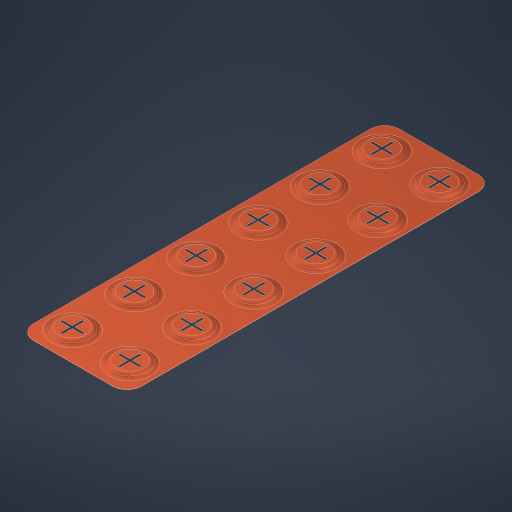
# Autodesk Inventor part: Bat_contacts_v1
Saved by Autodesk Inventor 2024.3 (Build 283343010, 343A)
## iProperties
Created: 2025-05-07
Part Number: Bat_contacts_v1
Material: Kupfer
Document SubType Name: Sheet Metal
Designer: David
Density: 8.94 g/cm^3
Appearance: Kupfer - satiniert
Sheet Metal Rule: Standard_mm
Author: David
Autodesk Inventor part; units mm, degrees
ref_plane "YZ Plane" through (0, 0, 0) normal (1, 0, 0) x (0, 1, 0)
ref_plane "XZ Plane" through (0, 0, 0) normal (0, 1, 0) x (-1, 0, 0)
ref_plane "XY Plane" through (0, 0, 0) normal (0, 0, 1) x (1, 0, 0)
sketch "Skizze1" plane through (0, 0, 0) normal (0, 0, 1) x (1, 0, 0)
  circle A0 centre (-20, 119.25) radius 9
  circle A1 centre (-20, 76.25) radius 9
  circle A2 centre (-20, 33.25) radius 9
  circle A3 centre (-20, 11.75) radius 9
  circle A4 centre (-20, 54.75) radius 9
  circle A5 centre (-20, 97.75) radius 9
  circle A6 centre (-40, 119.25) radius 9
  circle A7 centre (-40, 76.25) radius 9
  circle A8 centre (-40, 33.25) radius 9
  circle A9 centre (-40, 11.75) radius 9
  circle A10 centre (-40, 54.75) radius 9
  circle A11 centre (-40, 97.75) radius 9
  circle A12 centre (-20, 11.75) radius 9
  circle A13 centre (-20, 76.25) radius 9
  circle A14 centre (-20, 76.25) radius 9
  line L0 (-48.75, 129) -> (-11.25, 129)
  line L1 (-11.25, 129) -> (-11.25, 2)
  line L2 (-11.25, 2) -> (-48.75, 2)
  line L3 (-48.75, 2) -> (-48.75, 129)
  line L4 (-25, 16.75) -> (-15, 16.75)
  line L5 (-15, 16.75) -> (-15, 6.75)
  line L6 (-15, 6.75) -> (-25, 6.75)
  line L7 (-25, 6.75) -> (-25, 16.75)
  line L8 (-45, 16.75) -> (-35, 16.75)
  line L9 (-45, 6.75) -> (-45, 16.75)
  line L10 (-35, 6.75) -> (-45, 6.75)
  line L11 (-35, 16.75) -> (-35, 6.75)
  line L12 (-25, 38.25) -> (-15, 38.25)
  line L13 (-25, 28.25) -> (-25, 38.25)
  line L14 (-15, 28.25) -> (-25, 28.25)
  line L15 (-15, 38.25) -> (-15, 28.25)
  line L16 (-45, 38.25) -> (-35, 38.25)
  line L17 (-45, 28.25) -> (-45, 38.25)
  line L18 (-35, 28.25) -> (-45, 28.25)
  line L19 (-35, 38.25) -> (-35, 28.25)
  line L20 (-25, 59.75) -> (-15, 59.75)
  line L21 (-25, 49.75) -> (-25, 59.75)
  line L22 (-15, 49.75) -> (-25, 49.75)
  line L23 (-15, 59.75) -> (-15, 49.75)
  line L24 (-45, 59.75) -> (-35, 59.75)
  line L25 (-45, 49.75) -> (-45, 59.75)
  line L26 (-35, 49.75) -> (-45, 49.75)
  line L27 (-35, 59.75) -> (-35, 49.75)
  line L28 (-25, 81.25) -> (-15, 81.25)
  line L29 (-25, 71.25) -> (-25, 81.25)
  line L30 (-15, 71.25) -> (-25, 71.25)
  line L31 (-15, 81.25) -> (-15, 71.25)
  line L32 (-45, 81.25) -> (-35, 81.25)
  line L33 (-45, 71.25) -> (-45, 81.25)
  line L34 (-35, 71.25) -> (-45, 71.25)
  line L35 (-35, 81.25) -> (-35, 71.25)
  line L36 (-25, 102.75) -> (-15, 102.75)
  line L37 (-25, 92.75) -> (-25, 102.75)
  line L38 (-15, 92.75) -> (-25, 92.75)
  line L39 (-15, 102.75) -> (-15, 92.75)
  line L40 (-45, 102.75) -> (-35, 102.75)
  line L41 (-45, 92.75) -> (-45, 102.75)
  line L42 (-35, 92.75) -> (-45, 92.75)
  line L43 (-35, 102.75) -> (-35, 92.75)
  line L44 (-25, 124.25) -> (-15, 124.25)
  line L45 (-25, 114.25) -> (-25, 124.25)
  line L46 (-15, 114.25) -> (-25, 114.25)
  line L47 (-15, 124.25) -> (-15, 114.25)
  line L48 (-45, 124.25) -> (-35, 124.25)
  line L49 (-45, 114.25) -> (-45, 124.25)
  line L50 (-35, 114.25) -> (-45, 114.25)
  line L51 (-35, 124.25) -> (-35, 114.25)
  line L52 (13.75, 2) -> (41.25, 2)
  line L53 (46.25, 7) -> (46.25, 124)
  line L54 (41.25, 129) -> (13.75, 129)
  line L55 (8.75, 124) -> (8.75, 7)
  line L56 (14, 11.25) -> (17, 11.25)
  line L57 (17, 11.25) -> (17, 8.25)
  arc A15 (17, 8.25) -> (18, 8.25) centre (17.5, 8.25) ccw
  line L58 (18, 8.25) -> (18, 11.25)
  line L59 (18, 11.25) -> (21, 11.25)
  arc A16 (21, 11.25) -> (21, 12.25) centre (21, 11.75) ccw
  line L60 (21, 12.25) -> (18, 12.25)
  line L61 (18, 12.25) -> (18, 15.25)
  arc A17 (18, 15.25) -> (17, 15.25) centre (17.5, 15.25) ccw
  line L62 (17, 15.25) -> (17, 12.25)
  line L63 (17, 12.25) -> (14, 12.25)
  arc A18 (14, 12.25) -> (14, 11.25) centre (14, 11.75) ccw
  arc A19 (34, 12.25) -> (34, 11.25) centre (34, 11.75) ccw
  line L64 (37, 12.25) -> (34, 12.25)
  line L65 (34, 11.25) -> (37, 11.25)
  line L66 (41, 12.25) -> (38, 12.25)
  line L67 (38, 11.25) -> (41, 11.25)
  arc A20 (41, 11.25) -> (41, 12.25) centre (41, 11.75) ccw
  line L68 (37, 11.25) -> (37, 8.25)
  arc A21 (37, 8.25) -> (38, 8.25) centre (37.5, 8.25) ccw
  line L69 (38, 8.25) -> (38, 11.25)
  line L70 (38, 12.25) -> (38, 15.25)
  line L71 (37, 15.25) -> (37, 12.25)
  arc A22 (38, 15.25) -> (37, 15.25) centre (37.5, 15.25) ccw
  arc A23 (14, 33.75) -> (14, 32.75) centre (14, 33.25) ccw
  line L72 (17, 33.75) -> (14, 33.75)
  line L73 (14, 32.75) -> (17, 32.75)
  line L74 (21, 33.75) -> (18, 33.75)
  line L75 (18, 32.75) -> (21, 32.75)
  arc A24 (21, 32.75) -> (21, 33.75) centre (21, 33.25) ccw
  line L76 (17, 32.75) -> (17, 29.75)
  arc A25 (17, 29.75) -> (18, 29.75) centre (17.5, 29.75) ccw
  line L77 (18, 29.75) -> (18, 32.75)
  line L78 (18, 33.75) -> (18, 36.75)
  line L79 (17, 36.75) -> (17, 33.75)
  arc A26 (18, 36.75) -> (17, 36.75) centre (17.5, 36.75) ccw
  arc A27 (34, 33.75) -> (34, 32.75) centre (34, 33.25) ccw
  line L80 (37, 33.75) -> (34, 33.75)
  line L81 (34, 32.75) -> (37, 32.75)
  line L82 (41, 33.75) -> (38, 33.75)
  line L83 (38, 32.75) -> (41, 32.75)
  arc A28 (41, 32.75) -> (41, 33.75) centre (41, 33.25) ccw
  line L84 (37, 32.75) -> (37, 29.75)
  arc A29 (37, 29.75) -> (38, 29.75) centre (37.5, 29.75) ccw
  line L85 (38, 29.75) -> (38, 32.75)
  line L86 (38, 33.75) -> (38, 36.75)
  line L87 (37, 36.75) -> (37, 33.75)
  arc A30 (38, 36.75) -> (37, 36.75) centre (37.5, 36.75) ccw
  arc A31 (14, 55.25) -> (14, 54.25) centre (14, 54.75) ccw
  line L88 (17, 55.25) -> (14, 55.25)
  line L89 (14, 54.25) -> (17, 54.25)
  line L90 (21, 55.25) -> (18, 55.25)
  line L91 (18, 54.25) -> (21, 54.25)
  arc A32 (21, 54.25) -> (21, 55.25) centre (21, 54.75) ccw
  line L92 (17, 54.25) -> (17, 51.25)
  arc A33 (17, 51.25) -> (18, 51.25) centre (17.5, 51.25) ccw
  line L93 (18, 51.25) -> (18, 54.25)
  line L94 (18, 55.25) -> (18, 58.25)
  line L95 (17, 58.25) -> (17, 55.25)
  arc A34 (18, 58.25) -> (17, 58.25) centre (17.5, 58.25) ccw
  arc A35 (34, 55.25) -> (34, 54.25) centre (34, 54.75) ccw
  line L96 (37, 55.25) -> (34, 55.25)
  line L97 (34, 54.25) -> (37, 54.25)
  line L98 (41, 55.25) -> (38, 55.25)
  line L99 (38, 54.25) -> (41, 54.25)
  arc A36 (41, 54.25) -> (41, 55.25) centre (41, 54.75) ccw
  line L100 (37, 54.25) -> (37, 51.25)
  arc A37 (37, 51.25) -> (38, 51.25) centre (37.5, 51.25) ccw
  line L101 (38, 51.25) -> (38, 54.25)
  line L102 (38, 55.25) -> (38, 58.25)
  line L103 (37, 58.25) -> (37, 55.25)
  arc A38 (38, 58.25) -> (37, 58.25) centre (37.5, 58.25) ccw
  arc A39 (14, 76.75) -> (14, 75.75) centre (14, 76.25) ccw
  line L104 (17, 76.75) -> (14, 76.75)
  line L105 (14, 75.75) -> (17, 75.75)
  line L106 (21, 76.75) -> (18, 76.75)
  line L107 (18, 75.75) -> (21, 75.75)
  arc A40 (21, 75.75) -> (21, 76.75) centre (21, 76.25) ccw
  line L108 (17, 75.75) -> (17, 72.75)
  arc A41 (17, 72.75) -> (18, 72.75) centre (17.5, 72.75) ccw
  line L109 (18, 72.75) -> (18, 75.75)
  line L110 (18, 76.75) -> (18, 79.75)
  line L111 (17, 79.75) -> (17, 76.75)
  arc A42 (18, 79.75) -> (17, 79.75) centre (17.5, 79.75) ccw
  arc A43 (34, 76.75) -> (34, 75.75) centre (34, 76.25) ccw
  line L112 (37, 76.75) -> (34, 76.75)
  line L113 (34, 75.75) -> (37, 75.75)
  line L114 (41, 76.75) -> (38, 76.75)
  line L115 (38, 75.75) -> (41, 75.75)
  arc A44 (41, 75.75) -> (41, 76.75) centre (41, 76.25) ccw
  line L116 (37, 75.75) -> (37, 72.75)
  arc A45 (37, 72.75) -> (38, 72.75) centre (37.5, 72.75) ccw
  line L117 (38, 72.75) -> (38, 75.75)
  line L118 (38, 76.75) -> (38, 79.75)
  line L119 (37, 79.75) -> (37, 76.75)
  arc A46 (38, 79.75) -> (37, 79.75) centre (37.5, 79.75) ccw
  arc A47 (14, 98.25) -> (14, 97.25) centre (14, 97.75) ccw
  line L120 (17, 98.25) -> (14, 98.25)
  line L121 (14, 97.25) -> (17, 97.25)
  line L122 (21, 98.25) -> (18, 98.25)
  line L123 (18, 97.25) -> (21, 97.25)
  arc A48 (21, 97.25) -> (21, 98.25) centre (21, 97.75) ccw
  line L124 (17, 97.25) -> (17, 94.25)
  arc A49 (17, 94.25) -> (18, 94.25) centre (17.5, 94.25) ccw
  line L125 (18, 94.25) -> (18, 97.25)
  line L126 (18, 98.25) -> (18, 101.25)
  line L127 (17, 101.25) -> (17, 98.25)
  arc A50 (18, 101.25) -> (17, 101.25) centre (17.5, 101.25) ccw
  arc A51 (34, 98.25) -> (34, 97.25) centre (34, 97.75) ccw
  line L128 (37, 98.25) -> (34, 98.25)
  line L129 (34, 97.25) -> (37, 97.25)
  line L130 (41, 98.25) -> (38, 98.25)
  line L131 (38, 97.25) -> (41, 97.25)
  arc A52 (41, 97.25) -> (41, 98.25) centre (41, 97.75) ccw
  line L132 (37, 97.25) -> (37, 94.25)
  arc A53 (37, 94.25) -> (38, 94.25) centre (37.5, 94.25) ccw
  line L133 (38, 94.25) -> (38, 97.25)
  line L134 (38, 98.25) -> (38, 101.25)
  line L135 (37, 101.25) -> (37, 98.25)
  arc A54 (38, 101.25) -> (37, 101.25) centre (37.5, 101.25) ccw
  arc A55 (14, 119.75) -> (14, 118.75) centre (14, 119.25) ccw
  line L136 (17, 119.75) -> (14, 119.75)
  line L137 (14, 118.75) -> (17, 118.75)
  line L138 (21, 119.75) -> (18, 119.75)
  line L139 (18, 118.75) -> (21, 118.75)
  arc A56 (21, 118.75) -> (21, 119.75) centre (21, 119.25) ccw
  line L140 (17, 118.75) -> (17, 115.75)
  arc A57 (17, 115.75) -> (18, 115.75) centre (17.5, 115.75) ccw
  line L141 (18, 115.75) -> (18, 118.75)
  line L142 (18, 119.75) -> (18, 122.75)
  line L143 (17, 122.75) -> (17, 119.75)
  arc A58 (18, 122.75) -> (17, 122.75) centre (17.5, 122.75) ccw
  arc A59 (34, 119.75) -> (34, 118.75) centre (34, 119.25) ccw
  line L144 (37, 119.75) -> (34, 119.75)
  line L145 (34, 118.75) -> (37, 118.75)
  line L146 (41, 119.75) -> (38, 119.75)
  line L147 (38, 118.75) -> (41, 118.75)
  arc A60 (41, 118.75) -> (41, 119.75) centre (41, 119.25) ccw
  line L148 (37, 118.75) -> (37, 115.75)
  arc A61 (37, 115.75) -> (38, 115.75) centre (37.5, 115.75) ccw
  line L149 (38, 115.75) -> (38, 118.75)
  line L150 (38, 119.75) -> (38, 122.75)
  line L151 (37, 122.75) -> (37, 119.75)
  arc A62 (38, 122.75) -> (37, 122.75) centre (37.5, 122.75) ccw
  arc A63 (41.25, 2) -> (46.25, 7) centre (41.25, 7) ccw
  arc A64 (8.75, 7) -> (13.75, 2) centre (13.75, 7) ccw
  arc A65 (13.75, 129) -> (8.75, 124) centre (13.75, 124) ccw
  arc A66 (46.25, 124) -> (41.25, 129) centre (41.25, 124) ccw
  point P0 (0, 0)
  point P1 (-20, 6.75)
  point P2 (-15, 11.75)
  point P3 (-40, 6.75)
  point P4 (-35, 11.75)
  point P5 (-20, 28.25)
  point P6 (-15, 33.25)
  point P7 (-40, 28.25)
  point P8 (-35, 33.25)
  point P9 (-20, 49.75)
  point P10 (-15, 54.75)
  point P11 (-40, 49.75)
  point P12 (-35, 54.75)
  point P13 (-20, 71.25)
  point P14 (-15, 76.25)
  point P15 (-40, 71.25)
  point P16 (-35, 76.25)
  point P17 (-20, 92.75)
  point P18 (-15, 97.75)
  point P19 (-40, 92.75)
  point P20 (-35, 97.75)
  point P21 (-20, 114.25)
  point P22 (-15, 119.25)
  point P23 (-40, 114.25)
  point P24 (-35, 119.25)
  point P25 (8.75, 2)
  dimension "Abstandsgröße" = 0.5
  dimension "d0" = 10
  dimension "d1" = 10
  dimension "d4" = 20
  dimension "d7" = 21.5
  dimension "d11" = 9.75
  dimension "d12" = 9.75
  dimension "d13" = 8.75
  dimension "d14" = 8.75
  dimension "d15" = 20
  dimension "d16" = 1
  dimension "d17" = 7
  dimension "d18" = 8.75
  dimension "d21" = 20
  dimension "d24" = 21.5
  dimension "d27" = 5
  dimension "d28" = 8.75
  constraints: 304 end point, 104 point on circle, 98 point on line, 67 centre point, 15 tangent, 8 parallel, 8 perpendicular, 6 horizontal, 4 equal radius, 4 horizontal alignment, 2 collinear, 2 midpoint, 2 vertical, 1 vertical alignment, 428 other
  measures "d0" distance of L4.end L5.end
  measures "d1" distance of L4.start L4.end
  measures "d4" distance of L4.start L8.start
  measures "d7" distance of L4.start L12.start
  measures "d11" distance from line of L0 A0.centre
  measures "d12" distance from line of A3.centre L2
  measures "d13" distance from line of L3 A6.centre
  measures "d14" distance from line of L1 A0.centre
  measures "d15" distance between parallel lines of L1 L55
  measures "d16" distance between parallel lines of L61 L62
  measures "d17" distance of A16.centre A18.centre
  measures "d18" distance from line of L55 A15.centre
  measures "d21" distance of L63.end L64.end
  measures "d24" distance of L63.end L72.end
  measures "d27" radius of A63
  measures "d28" distance from line of L53 A21.centre
extrude "Extrusion1" add sketch "Skizze1" along normal blind 10 contours A64 L55 A65 L54 A66 L53 A63 L52 | A18 L63 L62 A17 L61 L60 A16 L59 L58 A15 L57 L56 | L64 L71 A22 L70 L66 A20 L67 L69 A21 L68 L65 A19 | L72 L79 A26 L78 L74 A24 L75 L77 A25 L76 L73 A23 | L80 L87 A30 L86 L82 A28 L83 L85 A29 L84 L81 A27 | L88 L95 A34 L94 L90 A32 L91 L93 A33 L92 L89 A31 | L96 L103 A38 L102 L98 A36 L99 L101 A37 L100 L97 A35 | L104 L111 A42 L110 L106 A40 L107 L109 A41 L108 L105 A39 | L112 L119 A46 L118 L114 A44 L115 L117 A45 L116 L113 A43 | L120 L127 A50 L126 L122 A48 L123 L125 A49 L124 L121 A47 | L128 L135 A54 L134 L130 A52 L131 L133 A53 L132 L129 A51 | L136 L143 A58 L142 L138 A56 L139 L141 A57 L140 L137 A55 | L144 L151 A62 L150 L146 A60 L147 L149 A61 L148 L145 A59
sketch "Skizze2" plane through (0, 0, 10) normal (0, 0, 1) x (1, 0, 0)
  circle A0 centre (17.5, 11.75) radius 6.5
  point P0 (0, 0)
  point P1 (14, 11.75)
  point P2 (17.5, 8.25)
  dimension "d32" = 13
  constraints: 1 centre point, 1 horizontal alignment, 1 vertical alignment
  measures "d32" diameter of A0
extrude "Extrusion2" add sketch "Skizze2" along normal blind 1
fillet "Rundung1" radius 2 2 edges at (11, 11.75, 11) (11, 11.75, 10)
pattern_linear "Rechteckige Anordnung1" count 2 spacing 20 along (1, 0, 0) count 6 spacing 21.5 along (0, 1, 0) of "Extrusion2", "Rundung1"
shell "Wandung1" thickness 0.15 removed faces 9 at (44.9153, 127.4009, 6.6667) at (41.6237, 2.014, 3.3333) at (32.0833, 129, 3.3333) at (22.9167, 2, 3.3333) at (8.764, 124.3737, 6.6667) at (11.25, 2.6699, 6.6667) at (8.75, 85, 3.3333) at (46.25, 46, 3.3333) at (33.75, 46, 0)
extrude "Ausschneiden1" cut sketch "Skizze1" along normal up to surface (11 mm away) contours A18 L63 L62 A17 L61 L60 A16 L59 L58 A15 L57 L56 | L64 L71 A22 L70 L66 A20 L67 L69 A21 L68 L65 A19 | L72 L79 A26 L78 L74 A24 L75 L77 A25 L76 L73 A23 | L80 L87 A30 L86 L82 A28 L83 L85 A29 L84 L81 A27 | L88 L95 A34 L94 L90 A32 L91 L93 A33 L92 L89 A31 | L96 L103 A38 L102 L98 A36 L99 L101 A37 L100 L97 A35 | L104 L111 A42 L110 L106 A40 L107 L109 A41 L108 L105 A39 | L112 L119 A46 L118 L114 A44 L115 L117 A45 L116 L113 A43 | L120 L127 A50 L126 L122 A48 L123 L125 A49 L124 L121 A47 | L128 L135 A54 L134 L130 A52 L131 L133 A53 L132 L129 A51 | L136 L143 A58 L142 L138 A56 L139 L141 A57 L140 L137 A55 | L144 L151 A62 L150 L146 A60 L147 L149 A61 L148 L145 A59
equation "\"Abstandsgröße\" = Stärke"
equation "\"d1\" = d0"
equation "\"d12\" = d11"
equation "\"d13\" = d14"
equation "\"d18\" = d14"
equation "\"d21\" = d4"
equation "\"d24\" = d7"
equation "\"d28\" = d18"
equation "\"d38\" = d4"
equation "\"d41\" = d7"
equation "\"d44\" = Stärke"
equation "\"Biegeradius\" = Stärke"
equation "\"BreiteBiegungsfreistellung\" = Stärke"
equation "\"TiefeBiegungsfreistellung\" = 0.5 * Stärke"
equation "\"GrößeEckenfreistellung\" = 4 * Stärke"
equation "\"MinimalRest\" = 2 * Stärke"
equation "\"Übergangsradius\" = Biegeradius"
equation "\"JacobiRadiusGröße\" = Biegeradius"
equation "\"d43\" = Stärke"
equation "\"Stärke\" = 0.5"
